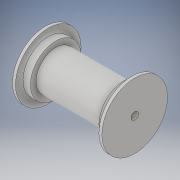
# Autodesk Inventor part: weel 2.2
Saved by Autodesk Inventor 2018.2 (Build 222227000, 227)
## iProperties
Created: 2018-01-27
Part Number: weel 2.2
Material: Generic
Document SubType Name: Modeling
Designer: MIABo
Density: 1 g/cm^3
Appearance: Default
Author: MIABo
Autodesk Inventor part; units mm, degrees
ref_plane "YZ Plane" through (0, 0, 0) normal (1, 0, 0) x (0, 1, 0)
ref_plane "XZ Plane" through (0, 0, 0) normal (0, 1, 0) x (-1, 0, 0)
ref_plane "XY Plane" through (0, 0, 0) normal (0, 0, 1) x (1, 0, 0)
sketch "Sketch1" plane through (0, 0, 0) normal (0, 0, 1) x (1, 0, 0)
  line L0 (-36.4853, -0.2751) -> (39.7147, -0.2751)
  line L1 (-36.4853, -0.2751) -> (-36.4853, 27.6649)
  line L2 (-36.4853, 27.6649) -> (-33.9453, 27.6649)
  arc A0 (-33.9453, 27.6649) -> (-33.9453, 21.3149) centre (-29.9798, 24.4899) ccw
  line L3 (-33.9453, 21.3149) -> (-27.5953, 21.3149)
  line L4 (-27.5953, 21.3149) -> (-27.5953, 16.5345)
  line L5 (39.7147, -0.2751) -> (39.7147, 27.6649)
  line L6 (39.7147, 27.6649) -> (37.1747, 27.6649)
  arc A1 (37.1747, 21.3149) -> (37.1747, 27.6649) centre (33.2091, 24.4899) ccw
  line L7 (37.1747, 21.3149) -> (30.8247, 21.3149)
  line L8 (30.8247, 21.3149) -> (30.8247, 16.5345)
  line L9 (-27.5953, 16.5345) -> (30.8247, 16.5345)
  point P0 (0, 0)
  dimension "d0" = 76.2
  dimension "d1" = 27.94
  dimension "d2" = 2.54
  dimension "d3" = 6.35
  dimension "d4" = 5.08
  dimension "d5" = 6.35
  constraints: 20 end point, 4 point on circle, 3 horizontal, 2 centre point, 2 vertical, 1 perpendicular
  measures "d0" distance of L0.start L0.end
  measures "d1" distance of L0.start L1.end
  measures "d2" distance of L1.end L2.end
  measures "d3" distance of L2.end L3.start
  measures "d4" radius of A0
  measures "d5" distance of L3.start L3.end
revolve "Revolution1" add sketch "Sketch1" angle 360 about axis through (-36.4853, -0.2751, 0) along (1, 0, 0)
sketch "Sketch2" plane through (0, 0, 0) normal (1, 0, 0) x (0, 1, 0)
  circle A0 centre (0, 0) radius 3.175
  circle A1 centre (0, 0) radius 3.175
  constraints: 2 centre point, 2 coincident, 1 concentric
sketch "Sketch3" plane through (-36.4853, -0.2751, 0) normal (-1, 0, 0) x (0, 0, 1)
  circle A0 centre (0, 0.2751) radius 3.175
  circle A1 centre (0, 0) radius 27.94 projected
  dimension "d9" = 6.35
  dimension "d10" = 25.0401
  constraints: 1 centre point
  measures "d9" diameter of A0
hole "Hole1" at (-36.4853, -0.2751, 0) direction (1, 0, 0) diameter 6.35 end through all both
sketch "Sketch4" plane through (-36.4853, -0.2751, 0) normal (-1, 0, 0) x (0, 0, 1)
  point P0 (0, 0.2751)
sketch "Sketch5" plane through (-36.4853, -0.2751, 0) normal (-1, 0, 0) x (0, 0, 1)
  point P0 (0, 0.2751)
sketch "Sketch6" plane through (39.7147, -0.2751, 0) normal (1, 0, 0) x (0, 0, -1)
  point P0 (0, 0.2751)
sketch "Sketch7" plane through (0, 0, 0) normal (1, 0, 0) x (0, 1, 0)
  point P0 (0, 0)
body "Solid1"
